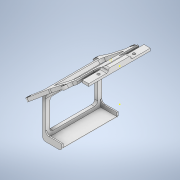
# Autodesk Inventor part: batteryBracket
Saved by Autodesk Inventor 2022 (Build 260153000, 153)
## iProperties
Created: 2022-04-12
Part Number: batteryBracket
Material: PLA Plastic
Document SubType Name: Modeling
Designer: Dahway
Mass: 20.6888 g
Surface Area: 158.166 cm^2
Volume: 20.6888 cm^3
Density: 1 g/cm^3
Appearance: PLA
Author: Dahway
Autodesk Inventor part; units mm, degrees
ref_plane "YZ Plane" through (0, 0, 0) normal (1, 0, 0) x (0, 1, 0)
ref_plane "XZ Plane" through (0, 0, 0) normal (0, 1, 0) x (-1, 0, 0)
ref_plane "XY Plane" through (0, 0, 0) normal (0, 0, 1) x (1, 0, 0)
sketch "Sketch1" plane through (0, 0, 0) normal (0, 1, 0) x (-1, 0, 0)
  line L0 (0, 0) -> (56, 0)
  line L1 (56, 0) -> (56, 75.4)
  line L2 (56, 75.4) -> (0, 75.4)
  line L3 (0, 75.4) -> (0, 0)
  dimension "d0" = 56
  dimension "d1" = 75.4
  constraints: 8 end point, 2 parallel, 1 horizontal, 1 perpendicular
  measures "d0" distance of L2.end L1.end
  measures "d1" distance of L1.end L0.end
extrude "Extrusion1" add sketch "Sketch1" along normal blind 40.7
sketch "Sketch2" plane through (0, 0, 0) normal (0, -1, 0) x (1, 0, 0)
  line L0 (0, 75.4) -> (0, 0) projected
  line L1 (-56, 75.4) -> (0, 75.4) projected
  line L2 (0, 0) -> (-7.8, 0)
  line L3 (-7.8, 0) -> (-7.8, 75.4)
  line L4 (-7.8, 75.4) -> (0, 75.4)
  line L5 (0, 75.4) -> (0, 0)
  dimension "d4" = 7.8
  constraints: 8 end point, 2 parallel, 1 horizontal, 1 perpendicular, 1 point on line
  measures "d4" distance of L3.end L4.end
extrude "Extrusion2" cut sketch "Sketch2" against normal blind 37.7
ref_plane "Work Plane1" through (0, 40.7, 37.7) normal (0, 0, -1) x (-1, 0, 0)
sketch "Sketch4" plane through (0, 37.7, 0) normal (0, -1, 0) x (1, 0, 0)
  circle A0 centre (-4, 3.7) radius 1.5
  circle A1 centre (-4, 6.5) radius 1.5
  line L0 (-5.5, 3.7) -> (-5.5, 6.5)
  line L1 (-2.5, 3.7) -> (-2.5, 6.5)
  line L2 (0, 0) -> (-7.8, 0) projected
  line L3 (0, 75.4) -> (0, 0) projected
  dimension "d17" = 3
  dimension "d18" = 3
  dimension "d19" = 3.7
  dimension "d20" = 4
  dimension "d21" = 2.8
  constraints: 4 end point, 4 point on circle, 2 centre point, 2 tangent, 1 parallel, 1 vertical
  measures "d17" diameter of A0
  measures "d18" diameter of A1
  measures "d19" distance from line of L2 A0.centre
  measures "d20" distance from line of L3 A0.centre
  measures "d21" distance of A1.centre A0.centre
extrude "Extrusion4" add sketch "Sketch4" along normal blind 3
fillet "Fillet1" radius 1 4 edges at (-4, 34.7, 2.2) (-2.5, 34.7, 5.1) (-4, 34.7, 8) (-5.5, 34.7, 5.1)
mirror "Mirror2" about plane through (0, 40.7, 37.7) normal (0, 0, -1) of "Extrusion4", "Fillet1"
sketch "Sketch5" plane through (0, 40.7, 0) normal (0, 0, -1) x (-1, 0, 0)
  line L0 (7.8, -3) -> (0, -3) projected
  line L1 (56, -40.7) -> (56, 0) projected
  line L2 (7.8, -3) -> (56, -40.7)
  line L3 (7.8, -3) -> (7.8, -40.7) projected
  line L4 (56, -40.7) -> (7.8, -40.7)
  line L5 (7.8, -40.7) -> (7.8, -3)
  line L6 (0, 0) -> (56, 0) projected
  line L7 (10.1465, 0) -> (56, -35.8647)
  line L8 (56, 0) -> (56, -35.8647)
  line L9 (10.1465, 0) -> (56, 0)
  point P0 (0, -40.7)
  dimension "d25" = 58.2136
  constraints: 12 end point, 2 point on line, 1 horizontal, 1 perpendicular, 1 vertical
  measures "d25" distance of L7.start L7.end
extrude "Extrusion5" cut sketch "Sketch5" against normal up to surface (75.4 mm away)
sketch "Sketch6" plane through (0, 37.7, 0) normal (0, 0, -1) x (-1, 0, 0)
  line L0 (7.8, 0) -> (56, -37.7) projected
  line L1 (56, -37.7) -> (56, -32.8647) projected
  line L2 (56, -32.8647) -> (10.1465, 3) projected
  line L3 (56, -37.7) -> (59.809, -37.7)
  line L4 (59.809, -37.7) -> (59.809, -35.8439)
  line L5 (59.809, -35.8439) -> (56, -32.8647)
  point P0 (0, -37.7)
  dimension "d32" = 3.809
  constraints: 6 end point, 1 collinear, 1 horizontal, 1 perpendicular
  measures "d32" distance of L0.end L3.end
extrude "Extrusion6" add sketch "Sketch6" against normal up to surface (75.4 mm away) fills toward (57.9045, -37.65) open curves L3 L4 L5
sketch "Sketch7" plane through (-59.809, 0, 0) normal (0, -1, 0) x (1, 0, 0)
  line L0 (0, 0) -> (49.6625, 0) projected
  line L1 (3.809, 0) -> (3.809, 75.4) projected
  line L2 (0, 0) -> (3.809, 0)
  line L3 (3.809, 0) -> (3.809, 75.4)
  line L4 (3.809, 75.4) -> (0, 75.4)
  line L5 (0, 75.4) -> (0, 0)
  point P0 (59.809, 0)
  constraints: 8 end point, 2 parallel, 1 horizontal, 1 perpendicular
extrude "Extrusion7" add sketch "Sketch7" along normal blind 50.5
sketch "Sketch8" plane through (-56, 0, 75.4) normal (1, 0, 0) x (0, 0, -1)
  line L0 (75.4, -50.5) -> (0, -50.5) projected
  line L1 (75.4, -50.5) -> (75.4, 1.8561) projected
  line L2 (0, -50.5) -> (75.4, -50.5)
  line L3 (75.4, -50.5) -> (75.4, -47.5)
  line L4 (75.4, -47.5) -> (0, -47.5)
  line L5 (0, -47.5) -> (0, -50.5)
  line L6 (4.8, -47.5) -> (3.3, -47.5)
  line L7 (3.3, -47.5) -> (3.3, -43)
  line L8 (3.3, -43) -> (4.8, -43)
  line L9 (4.8, -43) -> (4.8, -47.5)
  line L10 (0, 0) -> (0, -50.5) projected
  line L11 (37.7, -47.5) -> (37.7, -35.8022)
  line L12 (72.1, -47.5) -> (72.1, -43)
  line L13 (72.1, -43) -> (70.6, -43)
  line L14 (70.6, -43) -> (70.6, -47.5)
  point P0 (75.4, 0)
  point P1 (3.3, -47.5)
  dimension "d36" = 3
  dimension "d37" = 1.5
  dimension "d38" = 4.5
  dimension "d39" = 3.3
  constraints: 24 end point, 4 parallel, 4 symmetric about line, 2 horizontal, 2 perpendicular, 2 point on line, 1 midpoint, 1 vertical
  measures "d36" distance of L3.end L2.end
  measures "d37" distance of L7.end L8.end
  measures "d38" distance of L6.end L7.end
  measures "d39" distance between parallel lines of L10 L7
extrude "Extrusion8" add sketch "Sketch8" along normal blind 20
sketch "Sketch10" plane through (0, 37.7, 0) normal (0, -1, 0) x (1, 0, 0)
  line L0 (-7.8, 0) -> (-7.8, 75.4) projected
  line L1 (-7.8, 75.4) -> (-14.2, 75.4)
  line L2 (-14.2, 75.4) -> (-14.2, 51.5)
  line L3 (-14.2, 51.5) -> (-7.8, 51.5)
  line L4 (-7.8, 51.5) -> (-7.8, 75.4)
  line L5 (0, 0) -> (-10.1465, 0) projected
  line L6 (-7.8, 0) -> (-14.2, 0)
  line L7 (-14.2, 0) -> (-14.2, 23.9)
  line L8 (-14.2, 23.9) -> (-7.8, 23.9)
  line L9 (-7.8, 23.9) -> (-7.8, 0)
  dimension "d48" = 6.4
  dimension "d49" = 23.9
  dimension "d50" = 6.4
  dimension "d51" = 23.9
  constraints: 16 end point, 4 parallel, 2 horizontal, 2 perpendicular, 2 point on line
  measures "d48" distance of L3.end L2.end
  measures "d49" distance of L2.end L1.end
  measures "d50" distance of L7.end L8.end
  measures "d51" distance of L6.end L7.end
extrude "Extrusion10" cut sketch "Sketch10" along normal mid plane 10
sketch "Sketch13" plane through (-59.809, -50.5, 75.4) normal (0, 0, 1) x (1, 0, 0)
  line L0 (23.809, 0) -> (23.809, 3) projected
  line L1 (0, 0) -> (0, 52.3561) projected
  line L2 (23.809, 0) -> (0, 0)
  line L3 (0, 0) -> (0, 3)
  line L4 (0, 3) -> (23.809, 3)
  line L5 (23.809, 3) -> (23.809, 0)
  line L6 (0, 52.3561) -> (45.609, 88.0295) projected
  line L7 (0, 3) -> (3.809, 3)
  line L8 (3.809, 3) -> (3.809, 55.3353)
  line L9 (3.809, 55.3353) -> (0, 55.3353)
  line L10 (0, 55.3353) -> (0, 3)
  point P0 (59.809, 50.5)
  point P1 (41.9071, 85.134)
  point P2 (3.809, 3)
  dimension "d68" = 3
  dimension "d69" = 3.809
  constraints: 16 end point, 4 parallel, 2 horizontal, 2 perpendicular, 2 point on line
  measures "d68" distance of L2.end L3.end
  measures "d69" distance of L9.end L8.end
extrude "Extrusion12" cut sketch "Sketch13" against normal up to surface (3.3 mm away) contours L2 L1 L4 L0 | L4 L1 L6 L8
mirror "Mirror4" about plane through (0, 40.7, 37.7) normal (0, 0, -1) of "Extrusion12"
sketch "Sketch14" plane through (-59.809, 1.8561, 72.1) normal (-0.6160879, 0.7876774, 0) x (0.7876774, 0.6160879, 0)
  line L0 (46.203, 72.1) -> (39.353, 72.1)
  line L1 (39.353, 72.1) -> (39.353, 78.95)
  line L2 (39.353, 78.95) -> (46.203, 78.95)
  line L3 (46.203, 78.95) -> (46.203, 72.1)
  line L4 (53.2033, 72.1) -> (53.2033, 44.5) projected
  line L5 (54.9336, 72.1) -> (1.8568, 72.1) projected
  line L6 (4.8357, 72.1) -> (57.9031, 72.1) projected
  circle A0 centre (-12.322, 75.525) radius 3.425
  line L7 (0, 68.8) -> (0, 0) projected
  line L8 (0, 68.8) -> (-13.1797, 72.2091)
  line L9 (-11.4613, 78.8401) -> (15.2565, 78.8401) construction
  line L10 (-11.4613, 78.8401) -> (14.4982, 72.1)
  line L11 (14.4982, 72.1) -> (4.8357, 72.1)
  line L12 (4.8357, 72.1) -> (4.8357, 68.8) projected
  line L13 (4.8357, 68.8) -> (0, 68.8)
  point P0 (45.9667, 72.1)
  point P1 (42.778, 75.525)
  dimension "d73" = 7.0003
  dimension "d74" = 6.85
  dimension "d75" = 3.425
  dimension "d76" = 3.425
  dimension "d79" = 6.85
  dimension "d80" = 6.85
  dimension "d81" = 3.425
  dimension "d82" = 55.1
  dimension "d84" = 9.6625
  constraints: 18 end point, 3 parallel, 2 horizontal, 2 perpendicular, 2 point on circle, 2 tangent, 1 centre point, 1 collinear, 1 point on line
  measures "d73" distance between parallel lines of L4 L3
  measures "d74" distance of L1.end L2.end
  measures "d75" distance from line of L2 point (42.778, 75.525)
  measures "d76" distance from line of L3 point (42.778, 75.525)
  measures "d79" distance between parallel lines of L5 L2
  measures "d80" diameter of A0
  measures "d81" distance from line of L5 A0.centre
  measures "d82" distance of A0.centre point (42.778, 75.525)
  measures "d84" distance of L6.start L10.end
extrude "Extrusion13" add sketch "Sketch14" against normal up to surface (3.8087 mm away)
mirror "Mirror5" about plane through (0, 40.7, 37.7) normal (0, 0, -1) of "Extrusion13"
ref_plane "Work Plane3" through (-17.9019, 34.634, 27.6) normal (-0.6160879, 0.7876774, 0) x (0.7876774, 0.6160879, 0)
sketch "Sketch15" plane through (-17.9019, 34.634, 27.6) normal (-0.6160879, 0.7876774, 0) x (0.7876774, 0.6160879, 0)
  line L0 (-7.0003, 27.6) -> (-7.0003, 34.45) projected
  line L1 (-7.0003, 34.45) -> (-13.8503, 34.45) projected
  arc A0 (-64.6646, 34.3401) -> (-66.383, 27.7091) centre (-65.5253, 31.025) ccw projected
  arc A1 (-66.383, -47.9091) -> (-64.6646, -54.5401) centre (-65.5253, -51.225) ccw projected
  line L2 (-7.0003, -47.8) -> (-7.0003, -54.65) projected
  line L3 (-7.0003, -54.65) -> (-13.8503, -54.65) projected
  point P0 (-7.2366, 27.6)
  point P1 (-10.4253, 31.025)
  point P2 (-10.4253, -51.225)
  dimension "d87" = 3.425
  dimension "d88" = 3.425
  dimension "d89" = 3.425
  dimension "d90" = 3.425
  constraints: 2 coincident
  measures "d87" distance from line of L0 point (-10.425, 31.025)
  measures "d88" distance from line of L1 point (-10.425, 31.025)
  measures "d89" distance from line of L2 point (-10.425, -51.225)
  measures "d90" distance from line of point (-10.425, -51.225) L3
hole "Hole1" at (-26.1137, 28.2111, -3.425) at (-69.5148, -5.7354, -3.425) at (-69.5148, -5.7354, 78.825) at (-26.1137, 28.2111, 78.825) direction (0.6160879, -0.7876774, 0) diameter 3.5 end through all
ref_plane "Work Plane2" through (-17.9019, 34.634, 27.6) normal (-0.6160879, 0.7876774, 0) x (0.7876774, 0.6160879, 0)
sketch "Sketch16" plane through (-17.9019, 34.634, 27.6) normal (-0.6160879, 0.7876774, 0) x (0.7876774, 0.6160879, 0)
  line L0 (-13.8503, -47.8) -> (-38.7051, -47.8) projected
  line L1 (0, -20.2) -> (0, -47.8) projected
  line L2 (-43.2032, 19.6) -> (-6.2032, 19.6)
  line L3 (-6.2032, 19.6) -> (-6.2032, -39.8)
  line L4 (-6.2032, -39.8) -> (-43.2032, -39.8)
  line L5 (-43.2032, -39.8) -> (-43.2032, 19.6)
  line L6 (-43.2032, 19.6) -> (-6.2032, -39.8) construction
  line L7 (-6.2032, 19.6) -> (-43.2032, -39.8) construction
  line L8 (4.6998, -47.8) -> (4.6998, -23.9) projected
  point P0 (-7.2366, 27.6)
  point P1 (-24.7032, -10.1)
  dimension "d98" = 37.7
  dimension "d100" = 37
  dimension "d101" = 59.4
  dimension "d105" = 29.403
  constraints: 12 end point, 2 midpoint, 2 parallel, 1 horizontal, 1 perpendicular
  measures "d98" distance from line of L0 point (-24.703, -10.1)
  measures "d100" distance of L3.end L4.end
  measures "d101" distance of L2.end L3.end
  measures "d105" distance from line of point (-24.703, -10.1) L8
extrude "Extrusion14" cut sketch "Sketch16" against normal up to surface (3.8087 mm away)
fillet "Fillet4" radius 4 4 edges at (-21.6148, 29.3123, 8) (-50.7589, 6.517, 8) (-21.6148, 29.3123, 67.4) (-50.7589, 6.517, 67.4)
sketch "Sketch17" plane through (-59.809, -50.5, 3.3) normal (-1, 0, 0) x (0, 0, 1)
  line L0 (0, 52.3561) -> (0, 0) projected
  line L1 (68.8, 0) -> (0, 0) projected
  line L2 (5, 44.5) -> (63.8, 44.5)
  line L3 (63.8, 44.5) -> (63.8, 7.5)
  line L4 (63.8, 7.5) -> (5, 7.5)
  line L5 (5, 7.5) -> (5, 44.5)
  line L6 (5, 44.5) -> (63.8, 7.5) construction
  line L7 (63.8, 44.5) -> (5, 7.5) construction
  point P0 (-3.3, 50.5)
  point P1 (34.4, 26)
  dimension "d107" = 34.4
  dimension "d108" = 26
  dimension "d109" = 58.8
  dimension "d110" = 37
  constraints: 12 end point, 2 midpoint, 2 parallel, 1 horizontal, 1 perpendicular
  measures "d107" distance from line of L0 point (34.4, 26)
  measures "d108" distance from line of L1 point (34.4, 26)
  measures "d109" distance of L3.end L4.end
  measures "d110" distance of L2.end L3.end
extrude "Extrusion15" cut sketch "Sketch17" against normal up to surface (3.809 mm away)
fillet "Fillet5" radius 4 8 edges at (-57.9045, -43, 67.1) (-57.9045, -43, 8.3) (-57.9045, -6, 8.3) (-57.9045, -6, 67.1) (-59.809, -50.5, 37.7) (-56, -43, 4.05) (-56, -43, 71.35) (-36, -50.5, 37.7)
fillet "Fillet6" radius 10 3 edges at (-56, 0, 37.7) (-47.2158, 9.2883, 75.4) (-47.2158, 9.2883, 0)
fillet "Fillet7" radius 3.425 8 edges at (-27.6383, 24.601, -6.85) (-22.2427, 28.8212, -6.85) (-27.6383, 24.601, 0) (-22.2427, 28.8212, 0) (-22.2427, 28.8212, 82.25) (-27.6383, 24.601, 82.25) (-27.6383, 24.601, 75.4) (-22.2427, 28.8212, 75.4)
sketch "Sketch18" plane through (-10.1465, 40.7, 51.5) normal (0, 0, 1) x (1, 0, 0)
  line L0 (2.3465, -3) -> (2.3465, 0) projected
  line L1 (-4.0535, -8) -> (-4.0461, -8) projected
  line L2 (2.3465, -3) -> (-4.0461, -3)
  line L3 (-4.0461, -3) -> (-4.0461, -8)
  line L4 (-4.0461, -8) -> (2.3465, -8)
  line L5 (2.3465, -8) -> (2.3465, -3)
  line L6 (2.3465, -3) -> (-4.0461, -8) projected
  line L7 (2.3465, -3) -> (-4.0461, -8)
  point P0 (10.1465, -40.7)
  constraints: 10 end point, 3 equal length, 1 horizontal, 1 perpendicular
extrude "Extrusion16" add sketch "Sketch18" against normal up to surface (27.6 mm away) contours L5 L4 L6
fillet "Fillet8" radius 3.2 7 edges at (-14.2, 35.1148, 23.9) (-7.8, 35.2, 23.9) (-14.2, 35.1148, 51.5) (-7.8, 35.2, 51.5) (-7.8, 32.7, 37.7) (-7.8, 39.2, 23.9) (-7.8, 39.2, 51.5)
sketch "Sketch20" plane through (0, 40.7, 37.7) normal (0, 0, -1) x (-1, 0, 0)
  point P0 (0, -40.7)
  point P1 (0, 0)
  point P2 (10.1465, 0)
sketch "Sketch21" plane through (-7.8, 40.7, 23.9) normal (0, 0, -1) x (-1, 0, 0)
  line L0 (-7.8, 0) -> (0, 0) projected
  line L1 (-7.8, 0) -> (-7.8, 4)
  line L2 (-7.8, 4) -> (-2.7676, 4)
  line L3 (2.3465, 0) -> (0, 0) projected
  line L4 (-2.7676, 4) -> (2.3465, 0)
  line L5 (2.3465, 0) -> (6.4, -3.1705) projected
  point P0 (-7.8, -40.7)
  dimension "d121" = 4
  constraints: 6 end point, 1 collinear, 1 perpendicular, 1 vertical
  measures "d121" distance of L0.start L1.end
extrude "Extrusion17" add sketch "Sketch21" against normal up to surface (27.6 mm away)
fillet "Fillet9" radius 2 5 edges at (-5.0732, 40.7, 23.9) (-2.5162, 44.7, 23.9) (-2.5162, 44.7, 51.5) (-5.0732, 40.7, 51.5) (-5.0324, 44.7, 37.7)
fillet "Fillet10" radius 1 8 edges at (-14.2, 37.5295, 10.35) (-9.6997, 41.0494, 23.6239) (-10.5693, 40.3693, 23.8709) (-13.2627, 38.2626, 22.9627) (-13.2627, 38.2626, 52.4373) (-10.5693, 40.3693, 51.5291) (-9.6997, 41.0494, 51.7761) (-14.2, 37.5295, 65.05)
sketch "Sketch22" plane through (0, 40.7, 0) normal (0, 1, 0) x (1, 0, 0)
  line L0 (-7.8, -75.4) -> (0, -75.4) projected
  line L1 (-7.8, -54.7) -> (-7.8, -75.4) projected
  line L2 (0, 0) -> (-7.8, 0) projected
  point P0 (-4, -59.3)
  point P1 (-3.9, -16.1)
  dimension "d126" = 16.1
  dimension "d127" = 3.8
  dimension "d128" = 16.1
  measures "d126" distance from line of L0 point (-4, -59.3)
  measures "d127" distance from line of L1 point (-4, -59.3)
  measures "d128" distance from line of L2 point (-3.9, -16.1)
hole "Hole2" at (-4, 40.7, 59.3) at (-3.9, 40.7, 16.1) direction (0, -1, 0) diameter 3.15 end through all
equation "\"d85\" = d80"
body "Solid1"
